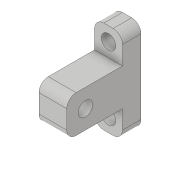
# Autodesk Inventor part: FTC Piv moount
Saved by Autodesk Inventor 2018 (Build 220112000, 112)
## iProperties
Created: 2017-12-20
Part Number: FTC Piv moount
Material: Generic
Document SubType Name: Modeling
Designer: dsayers
Density: 1 g/cm^3
Appearance: Default
Author: dsayers
Autodesk Inventor part; units mm, degrees
ref_plane "YZ Plane" through (0, 0, 0) normal (1, 0, 0) x (0, 1, 0)
ref_plane "XZ Plane" through (0, 0, 0) normal (0, 1, 0) x (-1, 0, 0)
ref_plane "XY Plane" through (0, 0, 0) normal (0, 0, 1) x (1, 0, 0)
sketch "Sketch1" plane through (0, 0, 0) normal (0, 0, 1) x (1, 0, 0)
  line L0 (0, 0) -> (9.525, 0)
  line L1 (9.525, 0) -> (9.525, 31.75)
  line L2 (9.525, 31.75) -> (0, 31.75)
  line L3 (0, 31.75) -> (0, 0)
  dimension "d0" = 9.525
  dimension "d1" = 31.75
  constraints: 8 end point, 2 parallel, 1 horizontal, 1 perpendicular
  measures "d0" distance of L1.end L2.end
  measures "d1" distance of L0.end L1.end
extrude "Extrusion1" add sketch "Sketch1" along normal blind 25.4
sketch "Sketch2" plane through (9.525, 0, 0) normal (1, 0, 0) x (0, 0, -1)
  line L0 (-25.4, 0) -> (-25.4, 31.75) projected
  line L1 (-25.4, 31.75) -> (-6.35, 31.75)
  line L2 (-6.35, 31.75) -> (-6.35, 22.225)
  line L3 (-6.35, 22.225) -> (-25.4, 22.225)
  line L4 (-25.4, 22.225) -> (-25.4, 31.75)
  line L5 (0, 0) -> (-25.4, 0) projected
  line L6 (-25.4, 0) -> (-6.35, 0)
  line L7 (-6.35, 0) -> (-6.35, 9.525)
  line L8 (-6.35, 9.525) -> (-25.4, 9.525)
  line L9 (-25.4, 9.525) -> (-25.4, 0)
  dimension "d4" = 9.525
  dimension "d5" = 9.525
  dimension "d6" = 19.05
  dimension "d7" = 19.05
  constraints: 16 end point, 4 parallel, 2 horizontal, 2 perpendicular
  measures "d4" distance of L6.end L7.end
  measures "d5" distance of L1.end L2.end
  measures "d6" distance of L2.end L3.end
  measures "d7" distance of L7.end L8.end
extrude "Extrusion2" cut sketch "Sketch2" against normal blind 25.4
fillet "Fillet1" radius 3.175 4 edges at (9.525, 31.75, 3.175) (0, 31.75, 3.175) (9.525, 0, 3.175) (0, 0, 3.175)
fillet "Fillet2" radius 3.175 2 edges at (4.7625, 9.525, 25.4) (4.7625, 22.225, 25.4)
sketch "Sketch3" plane through (9.525, 3.175, 0) normal (1, 0, 0) x (0, 0, -1)
  line L0 (-22.225, 6.35) -> (-6.35, 6.35) projected
  line L1 (-6.35, 19.05) -> (-22.225, 19.05) projected
  line L2 (0, 0) -> (0, 25.4) projected
  point P0 (0, -3.175)
  point P1 (-19.05, 12.7)
  dimension "d12" = 6.35
  dimension "d13" = 6.35
  dimension "d14" = 19.05
  measures "d12" distance from line of L0 point (-19.05, 12.7)
  measures "d13" distance from line of L1 point (-19.05, 12.7)
  measures "d14" distance from line of L2 point (-19.05, 12.7)
hole "Hole1" at (9.525, 15.875, 19.05) direction (-1, 0, 0) diameter 4.9276 depth 25.4 tip angle 118 clearance for "Flat Head Machine Screw (82)" size "#8" standard "Ansi Unified Screw Threads"
sketch "Sketch4" plane through (0, 22.225, 6.35) normal (0, 0, 1) x (1, 0, 0)
  line L0 (0, 0) -> (0, 6.35) projected
  line L1 (9.525, 6.35) -> (9.525, 0) projected
  line L2 (0, -19.05) -> (0, -12.7) projected
  line L3 (9.525, -12.7) -> (9.525, -19.05) projected
  line L4 (6.35, -22.225) -> (3.175, -22.225) projected
  line L5 (3.175, 9.525) -> (6.35, 9.525) projected
  point P0 (0, -22.225)
  point P1 (4.7625, -17.4625)
  point P2 (4.7625, 4.7625)
  dimension "d22" = 4.7625
  dimension "d23" = 4.7625
  dimension "d24" = 4.7625
  dimension "d25" = 4.7625
  dimension "d26" = 4.7625
  dimension "d27" = 4.7625
  dimension "d28" = 22.225
  measures "d22" distance from line of L0 point (4.763, 4.763)
  measures "d23" distance from line of L1 point (4.763, 4.763)
  measures "d24" distance from line of L2 point (4.762, -17.462)
  measures "d25" distance from line of L3 point (4.762, -17.462)
  measures "d26" distance from line of L4 point (4.762, -17.462)
  measures "d27" distance from line of point (4.763, 4.763) L5
  measures "d28" distance of point (4.762, -17.462) point (4.763, 4.763)
hole "Hole2" at (4.7625, 4.7625, 6.35) at (4.7625, 26.9875, 6.35) direction (0, 0, -1) diameter 4.9276 depth 25.4 tip angle 118 clearance for "Flat Head Machine Screw (82)" size "#8" standard "Ansi Unified Screw Threads"
equation "\"d5\" = d4"
equation "\"d7\" = d6"
equation "\"d12\" = d13"
equation "\"d22\" = d23"
equation "\"d24\" = d25"
equation "\"d26\" = d27"
body "Solid1"
